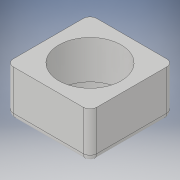
# Autodesk Inventor part: tail-rolley-polley
Saved by Autodesk Inventor 2019 (Build 230136000, 136)
## iProperties
Created: 2019-06-06
Part Number: tail-rolley-polley
Material: Generic
Document SubType Name: Modeling
Designer: Cole
Density: 1 g/cm^3
Appearance: Default
Author: Cole
Autodesk Inventor part; units mm, degrees
ref_plane "YZ Plane" through (0, 0, 0) normal (1, 0, 0) x (0, 1, 0)
ref_plane "XZ Plane" through (0, 0, 0) normal (0, 1, 0) x (-1, 0, 0)
sketch "Sketch1" plane through (0, 0, 0) normal (0, 1, 0) x (-1, 0, 0)
  line L0 (0, 0) -> (19.431, 0)
  line L1 (19.431, 0) -> (19.431, -19.431)
  line L2 (19.431, -19.431) -> (0, -19.431)
  line L3 (0, -19.431) -> (0, 0)
  dimension "d0" = 19.431
  dimension "d1" = 19.431
  constraints: 8 end point, 2 parallel, 1 horizontal, 1 perpendicular
  measures "d0" distance of L0.end L1.end
  measures "d1" distance of L1.end L2.end
extrude "Extrusion1" add sketch "Sketch1" along normal blind 10.922
ref_plane "Work Plane2" through (-19.431, 0, -9.7155) normal (0, 0, 1) x (1, 0, 0)
sketch "Sketch2" plane through (-19.431, 0, -9.7155) normal (0, 0, 1) x (1, 0, 0)
  arc A0 (9.7155, -5.2517) -> (16.9545, 1.9873) centre (9.7155, 1.9873) ccw
  line L0 (16.9545, 1.9873) -> (16.9545, 10.922)
  line L1 (19.431, 10.922) -> (0, 10.922) projected
  line L2 (9.7155, -5.3792) -> (9.7155, 10.922)
  line L3 (16.9545, 10.922) -> (9.7155, 10.922)
  point P0 (19.431, 0)
  dimension "d4" = 14.478
  constraints: 6 end point, 2 perpendicular, 2 point on circle, 2 point on line, 1 centre point, 1 midpoint
  measures "d4" diameter of A0
revolve "Revolution1" cut sketch "Sketch2" angle 360 about axis through (-9.7155, -5.3792, -9.7155) along (0, 1, 0)
fillet "Fillet1" radius 1.5875 2 edges at (-9.7155, 0, -19.431) (0, 0, -9.7155)
fillet "Fillet2" radius 1.5875 9 edges at (-19.431, 0, -8.9218) (-19.431, 0.465, -18.966) (-19.431, 6.2548, -19.431) (-0.465, 0.465, 0) (0, 6.2548, 0) (-10.5092, 0, 0) (-0.465, 0.465, -18.966) (0, 6.2548, -19.431) (-19.431, 5.461, 0)
equation "\"d1\" = d0"
body "Solid1"
